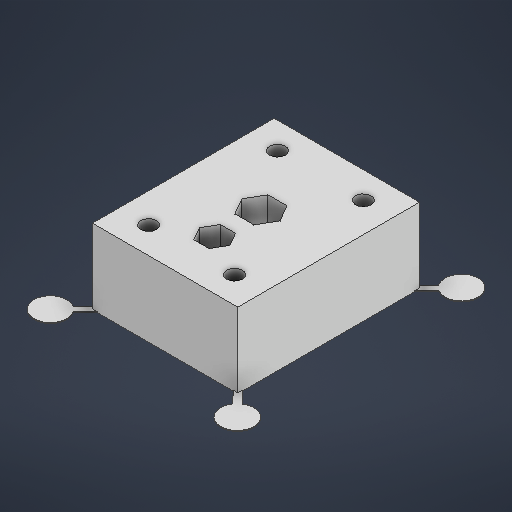
# Autodesk Inventor part: adapter-optical
Saved by Autodesk Inventor 2026.2 (Build 302298000, 298)
## iProperties
Created: 2026-05-22
Part Number: adapter-optical
Material: Generic
Document SubType Name: Modeling
Designer: mayhe
Density: 1 g/cm^3
Appearance: Default
Mass: 51.2124 g
Surface Area: 118.535 cm^2
Volume: 51.2124 cm^3
Author: mayhe
Autodesk Inventor part; units mm, degrees
ref_plane "YZ Plane" through (0, 0, 0) normal (1, 0, 0) x (0, 1, 0)
ref_plane "XZ Plane" through (0, 0, 0) normal (0, 1, 0) x (-1, 0, 0)
ref_plane "XY Plane" through (0, 0, 0) normal (0, 0, 1) x (1, 0, 0)
sketch "Sketch1" plane through (0, 0, 0) normal (1, 0, 0) x (0, 1, 0)
  line L0 (11.35, 27.5) -> (-11.35, 27.5)
  line L1 (-11.35, 27.5) -> (-11.35, -27.5)
  line L2 (-11.35, -27.5) -> (11.35, -27.5)
  line L3 (11.35, -27.5) -> (11.35, 27.5)
  line L4 (11.35, 27.5) -> (-11.35, -27.5) construction
  line L5 (-11.35, 27.5) -> (11.35, -27.5) construction
  point P0 (0, 0)
  dimension "d0" = 22.7
  dimension "d1" = 55
  constraints: 12 end point, 2 midpoint, 2 parallel, 1 horizontal, 1 perpendicular
  measures "d0" distance of L2.end L1.end
  measures "d1" distance of L1.end L0.end
extrude "Extrusion1" add sketch "Sketch1" along normal mid plane 44
sketch "Sketch4" plane through (-22, -11.35, 19.5) normal (0, 1, 0) x (1, 0, 0)
  circle A0 centre (9, 39) radius 2.375
  line L0 (0, 47) -> (44, 47) projected
  line L1 (0, -8) -> (0, 47) projected
  circle A1 centre (35, 39) radius 2.375
  circle A2 centre (9, 0) radius 2.375
  circle A3 centre (35, 0) radius 2.375
  line L2 (44, -8) -> (0, -8) projected
  point P0 (22, 19.5)
  dimension "d23" = 4.75
  dimension "d24" = 8
  dimension "d25" = 9
  dimension "d28" = 26
  dimension "d31" = 39
  dimension "d69" = 8
  constraints: 4 centre point, 1 horizontal, 1 vertical, 6 other
  measures "d23" diameter of A0
  measures "d24" distance from line of L0 A0.centre
  measures "d25" distance from line of L1 A0.centre
  measures "d28" distance of A0.centre A1.centre
  measures "d31" distance of A0.centre A2.centre
  measures "d69" distance from line of L2 A2.centre
hole "Event Camera mounting bolts" at (13, -11.35, -19.5) at (-13, -11.35, -19.5) at (-13, -11.35, 19.5) at (13, -11.35, 19.5) direction (0, 1, 0) diameter 4.75 depth 22.7 tip angle 118 counterbore diameter 7.7 counterbore depth 3
sketch "Sketch5" plane through (-22, -11.35, -27.5) normal (0, -1, 0) x (1, 0, 0)
  circle A0 centre (22, 40) radius 2
  circle A1 centre (22, 26) radius 2.5
  line L0 (44, 55) -> (0, 55) projected
  point P0 (22, 27.5)
  dimension "d41" = 4
  dimension "d42" = 5
  dimension "d43" = 14
  dimension "d44" = 15
  constraints: 2 centre point
  measures "d41" diameter of A0
  measures "d42" diameter of A1
  measures "d43" distance of A0.centre A1.centre
  measures "d44" distance from line of L0 A0.centre
hole "Small Hole" at (0, -11.35, 12.5) direction (0, 1, 0) diameter 5.75 depth 22.7 tip angle 118
hole "Big Hole" at (0, -11.35, -1.5) direction (0, 1, 0) diameter 6.75 depth 22.7 tip angle 118
sketch "Sketch6" plane through (-22, 11.35, 27.5) normal (0, 1, 0) x (1, 0, 0)
  circle A0 centre (22, 29) radius 3.375 projected
  circle A1 centre (22, 29) radius 5
  circle A2 centre (22, 15) radius 2.875 projected
  circle A3 centre (22, 15) radius 4
  line L0 (19.1132, 24) -> (16.2265, 29)
  line L1 (16.2265, 29) -> (19.1132, 34)
  line L2 (19.1132, 34) -> (24.8868, 34)
  line L3 (24.8868, 34) -> (27.7735, 29)
  line L4 (27.7735, 29) -> (24.8868, 24)
  line L5 (24.8868, 24) -> (19.1132, 24)
  line L6 (19.689, 11.0009) -> (17.3812, 15.0019)
  line L7 (17.3812, 15.0019) -> (19.6922, 19.0009)
  line L8 (19.6922, 19.0009) -> (24.311, 18.9991)
  line L9 (24.311, 18.9991) -> (26.6188, 14.9981)
  line L10 (26.6188, 14.9981) -> (24.3078, 10.9991)
  line L11 (24.3078, 10.9991) -> (19.689, 11.0009)
  point P0 (22, 27.5)
  point P1 (22, 24)
  point P2 (21.9984, 11)
  dimension "d59" = 10
  dimension "d60" = 8
  constraints: 24 end point, 4 coincident, 2 midpoint, 1 vertical alignment, 31 other
extrude "Big Hole Nut" cut sketch "Sketch6" against normal blind 8.5668 contours A0 | A1 | A1 L3 L4 | A1 L2 L3 | L4 L5 A1 | A1 L1 L2 | L5 L0 A1 | A1 L0 L1
extrude "Small Hole Nut" cut sketch "Sketch6" against normal blind 6.9668 contours A2 | A3 | A3 L9 L10 | A3 L8 L9 | L10 L11 A3 | A3 L7 L8 | L11 L6 A3 | A3 L6 L7
sketch "Sketch8" plane through (22, 11.35, -27.5) normal (0, 0, -1) x (-1, 0, 0)
  line L0 (-7.9257, -5.0636) -> (51.9257, -5.0636) construction
  line L1 (51.9257, -5.0636) -> (51.9257, -17.6364) construction
  line L2 (51.9257, -17.6364) -> (-7.9257, -17.6364) construction
  line L3 (-7.9257, -17.6364) -> (-7.9257, -5.0636) construction
  line L4 (24.8868, 0) -> (19.1132, 0) projected
  line L5 (22, 0) -> (22, -22.7)
  line L6 (44, -22.7) -> (0, -22.7) projected
  line L7 (44, 0) -> (0, 0) projected
  line L8 (7.086, -7.396) -> (7.086, -4.221)
  line L9 (7.086, -4.221) -> (9.2318, -4.221)
  line L10 (9.2318, -4.221) -> (9.2318, -4.8257)
  line L11 (9.2318, -4.8257) -> (7.8785, -4.8257)
  line L12 (7.8785, -4.8257) -> (7.8785, -5.384)
  line L13 (7.8785, -5.384) -> (9.1263, -5.384)
  line L14 (9.1263, -5.384) -> (9.1263, -5.9887)
  line L15 (9.1263, -5.9887) -> (7.8785, -5.9887)
  line L16 (7.8785, -5.9887) -> (7.8785, -6.7914)
  line L17 (7.8785, -6.7914) -> (9.2318, -6.7914)
  line L18 (9.2318, -6.7914) -> (9.2318, -7.396)
  line L19 (9.2318, -7.396) -> (7.086, -7.396)
  line L20 (11.9694, -5.0006) -> (11.1101, -7.396)
  line L21 (11.1101, -7.396) -> (10.2944, -7.396)
  line L22 (10.2944, -7.396) -> (9.4428, -5.0006)
  line L23 (9.4428, -5.0006) -> (10.2275, -5.0006)
  line L24 (10.2275, -5.0006) -> (10.719, -6.583)
  line L25 (10.719, -6.583) -> (11.2001, -5.0006)
  line L26 (11.2001, -5.0006) -> (11.9694, -5.0006)
  spline S0 degree 2 poles (13.4823, -7.4604) (12.803, -7.4604) (12.0801, -6.812) (12.0801, -6.2125) knots 0 0 0 1 2 2 2
  spline S1 degree 2 poles (12.0801, -6.2125) (12.0801, -5.6259) (12.7542, -4.926) (13.3614, -4.926) knots 0 0 0 1 2 2 2
  spline S2 degree 2 poles (13.3614, -4.926) (13.9094, -4.926) (14.4652, -5.5204) (14.4652, -6.071) knots 0 0 0 1 2 2 2
  line L27 (14.4652, -6.071) -> (14.4652, -6.3411)
  line L28 (14.4652, -6.3411) -> (12.8262, -6.3411)
  spline S3 degree 2 poles (12.8262, -6.3411) (12.8365, -6.5084) (12.9574, -6.7297) (13.0552, -6.7966) knots 0 0 0 1 2 2 2
  spline S4 degree 2 poles (13.0552, -6.7966) (13.1504, -6.8635) (13.4077, -6.9201) (13.5595, -6.9201) knots 0 0 0 1 2 2 2
  spline S5 degree 2 poles (13.5595, -6.9201) (13.6881, -6.9201) (13.9403, -6.8635) (14.0458, -6.8146) knots 0 0 0 1 2 2 2
  spline S6 degree 2 poles (14.0458, -6.8146) (14.1384, -6.776) (14.2928, -6.6808) (14.3417, -6.6448) knots 0 0 0 1 2 2 2
  line L29 (14.3417, -6.6448) -> (14.4214, -6.6448)
  line L30 (14.4214, -6.6448) -> (14.4214, -7.2623)
  spline S7 degree 2 poles (14.4214, -7.2623) (14.3288, -7.2983) (14.1796, -7.36) (14.0458, -7.3909) knots 0 0 0 1 2 2 2
  spline S8 degree 2 poles (14.0458, -7.3909) (13.9248, -7.4244) (13.6676, -7.4604) (13.4823, -7.4604) knots 0 0 0 1 2 2 2
  spline S9 degree 2 poles (13.7293, -5.8909) (13.7242, -5.6542) (13.5158, -5.4046) (13.3022, -5.4046) knots 0 0 0 1 2 2 2
  spline S10 degree 2 poles (13.3022, -5.4046) (13.0835, -5.4046) (12.8365, -5.667) (12.8236, -5.8909) knots 0 0 0 1 2 2 2
  line L31 (12.8236, -5.8909) -> (13.7293, -5.8909)
  line L32 (17.0896, -7.396) -> (16.3383, -7.396)
  line L33 (16.3383, -7.396) -> (16.3383, -6.2099)
  spline S11 degree 2 poles (16.3383, -6.2099) (16.3383, -6.0633) (16.3151, -5.7751) (16.2842, -5.7082) knots 0 0 0 1 2 2 2
  spline S12 degree 2 poles (16.2842, -5.7082) (16.2456, -5.6259) (16.1016, -5.5564) (15.978, -5.5564) knots 0 0 0 1 2 2 2
  spline S13 degree 2 poles (15.978, -5.5564) (15.888, -5.5564) (15.7002, -5.6259) (15.5947, -5.7005) knots 0 0 0 1 2 2 2
  line L34 (15.5947, -5.7005) -> (15.5947, -7.396)
  line L35 (15.5947, -7.396) -> (14.8485, -7.396)
  line L36 (14.8485, -7.396) -> (14.8485, -5.0006)
  line L37 (14.8485, -5.0006) -> (15.5947, -5.0006)
  line L38 (15.5947, -5.0006) -> (15.5947, -5.2657)
  spline S14 degree 2 poles (15.5947, -5.2657) (15.7774, -5.1113) (16.1247, -4.9363) (16.3357, -4.9363) knots 0 0 0 1 2 2 2
  spline S15 degree 2 poles (16.3357, -4.9363) (16.701, -4.9363) (17.0896, -5.3995) (17.0896, -5.8369) knots 0 0 0 1 2 2 2
  line L39 (17.0896, -5.8369) -> (17.0896, -7.396)
  spline S16 degree 2 poles (18.5587, -7.4424) (18.1033, -7.4424) (17.6865, -7.0667) (17.6865, -6.6396) knots 0 0 0 1 2 2 2
  line L40 (17.6865, -6.6396) -> (17.6865, -5.5204)
  line L41 (17.6865, -5.5204) -> (17.4009, -5.5204)
  line L42 (17.4009, -5.5204) -> (17.4009, -5.0006)
  line L43 (17.4009, -5.0006) -> (17.6865, -5.0006)
  line L44 (17.6865, -5.0006) -> (17.6865, -4.3162)
  line L45 (17.6865, -4.3162) -> (18.4326, -4.3162)
  line L46 (18.4326, -4.3162) -> (18.4326, -5.0006)
  line L47 (18.4326, -5.0006) -> (19.153, -5.0006)
  line L48 (19.153, -5.0006) -> (19.153, -5.5204)
  line L49 (19.153, -5.5204) -> (18.4326, -5.5204)
  line L50 (18.4326, -5.5204) -> (18.4326, -6.372)
  spline S17 degree 2 poles (18.4326, -6.372) (18.4326, -6.4981) (18.4378, -6.6859) (18.4686, -6.7605) knots 0 0 0 1 2 2 2
  spline S18 degree 2 poles (18.4686, -6.7605) (18.4995, -6.8351) (18.6513, -6.9226) (18.7954, -6.9226) knots 0 0 0 1 2 2 2
  spline S19 degree 2 poles (18.7954, -6.9226) (18.8572, -6.9226) (19.0501, -6.8712) (19.0887, -6.8506) knots 0 0 0 1 2 2 2
  line L51 (19.0887, -6.8506) -> (19.153, -6.8506)
  line L52 (19.153, -6.8506) -> (19.153, -7.3755)
  spline S20 degree 2 poles (19.153, -7.3755) (19.0321, -7.4063) (18.7594, -7.4424) (18.5587, -7.4424) knots 0 0 0 1 2 2 2
  spline S21 degree 2 poles (22.1479, -7.4578) (21.4327, -7.4578) (20.5939, -6.5933) (20.5939, -5.8111) knots 0 0 0 1 2 2 2
  spline S22 degree 2 poles (20.5939, -5.8111) (20.5939, -5.0573) (21.4352, -4.1593) (22.1505, -4.1593) knots 0 0 0 1 2 2 2
  spline S23 degree 2 poles (22.1505, -4.1593) (22.3383, -4.1593) (22.6419, -4.203) (22.7809, -4.2391) knots 0 0 0 1 2 2 2
  spline S24 degree 2 poles (22.7809, -4.2391) (22.8889, -4.2725) (23.1437, -4.3831) (23.2234, -4.4243) knots 0 0 0 1 2 2 2
  line L53 (23.2234, -4.4243) -> (23.2234, -5.1808)
  line L54 (23.2234, -5.1808) -> (23.1437, -5.1808)
  spline S25 degree 2 poles (23.1437, -5.1808) (23.0845, -5.1293) (22.9095, -4.9852) (22.7989, -4.9183) knots 0 0 0 1 2 2 2
  spline S26 degree 2 poles (22.7989, -4.9183) (22.6883, -4.8488) (22.4232, -4.7536) (22.2766, -4.7536) knots 0 0 0 1 2 2 2
  spline S27 degree 2 poles (22.2766, -4.7536) (22.1042, -4.7536) (21.8186, -4.8617) (21.6874, -4.9981) knots 0 0 0 1 2 2 2
  spline S28 degree 2 poles (21.6874, -4.9981) (21.569, -5.119) (21.4172, -5.5332) (21.4172, -5.8137) knots 0 0 0 1 2 2 2
  spline S29 degree 2 poles (21.4172, -5.8137) (21.4172, -6.1096) (21.5742, -6.5135) (21.7028, -6.637) knots 0 0 0 1 2 2 2
  spline S30 degree 2 poles (21.7028, -6.637) (21.8263, -6.758) (22.1299, -6.8635) (22.2817, -6.8635) knots 0 0 0 1 2 2 2
  spline S31 degree 2 poles (22.2817, -6.8635) (22.4387, -6.8635) (22.7243, -6.758) (22.8221, -6.6936) knots 0 0 0 1 2 2 2
  spline S32 degree 2 poles (22.8221, -6.6936) (22.9301, -6.6293) (23.0922, -6.4929) (23.1514, -6.4389) knots 0 0 0 1 2 2 2
  line L55 (23.1514, -6.4389) -> (23.2234, -6.4389)
  line L56 (23.2234, -6.4389) -> (23.2234, -7.1851)
  spline S33 degree 2 poles (23.2234, -7.1851) (23.136, -7.2262) (22.907, -7.3292) (22.7835, -7.3652) knots 0 0 0 1 2 2 2
  spline S34 degree 2 poles (22.7835, -7.3652) (22.6342, -7.4115) (22.3744, -7.4578) (22.1479, -7.4578) knots 0 0 0 1 2 2 2
  spline S35 degree 2 poles (24.9705, -7.1413) (24.8933, -7.2057) (24.7723, -7.3086) (24.6694, -7.36) knots 0 0 0 1 2 2 2
  spline S36 degree 2 poles (24.6694, -7.36) (24.5691, -7.4089) (24.3787, -7.4604) (24.2089, -7.4604) knots 0 0 0 1 2 2 2
  spline S37 degree 2 poles (24.2089, -7.4604) (23.8898, -7.4604) (23.4704, -7.0333) (23.4704, -6.7091) knots 0 0 0 1 2 2 2
  spline S38 degree 2 poles (23.4704, -6.7091) (23.4704, -6.4441) (23.684, -6.1147) (23.8847, -6.0195) knots 0 0 0 1 2 2 2
  spline S39 degree 2 poles (23.8847, -6.0195) (24.0879, -5.9218) (24.6514, -5.8446) (24.9756, -5.824) knots 0 0 0 1 2 2 2
  line L57 (24.9756, -5.824) -> (24.9756, -5.8111)
  spline S40 degree 2 poles (24.9756, -5.8111) (24.9756, -5.613) (24.6823, -5.4612) (24.389, -5.4612) knots 0 0 0 1 2 2 2
  spline S41 degree 2 poles (24.389, -5.4612) (24.2577, -5.4612) (23.9027, -5.5564) (23.7354, -5.631) knots 0 0 0 1 2 2 2
  line L58 (23.7354, -5.631) -> (23.6711, -5.631)
  line L59 (23.6711, -5.631) -> (23.6711, -5.0521)
  spline S42 degree 2 poles (23.6711, -5.0521) (23.7818, -5.0212) (24.2758, -4.9338) (24.5279, -4.9338) knots 0 0 0 1 2 2 2
  spline S43 degree 2 poles (24.5279, -4.9338) (25.1454, -4.9338) (25.7115, -5.3454) (25.7115, -5.7674) knots 0 0 0 1 2 2 2
  line L60 (25.7115, -5.7674) -> (25.7115, -7.396)
  line L61 (25.7115, -7.396) -> (24.9705, -7.396)
  line L62 (24.9705, -7.396) -> (24.9705, -7.1413)
  line L63 (24.9705, -6.7708) -> (24.9705, -6.2742)
  spline S44 degree 2 poles (24.9705, -6.2742) (24.7801, -6.2923) (24.5459, -6.3206) (24.4327, -6.3617) knots 0 0 0 1 2 2 2
  spline S45 degree 2 poles (24.4327, -6.3617) (24.3324, -6.3952) (24.2243, -6.5341) (24.2243, -6.6473) knots 0 0 0 1 2 2 2
  spline S46 degree 2 poles (24.2243, -6.6473) (24.2243, -6.8146) (24.407, -6.9406) (24.5845, -6.9406) knots 0 0 0 1 2 2 2
  spline S47 degree 2 poles (24.5845, -6.9406) (24.6823, -6.9406) (24.8881, -6.8506) (24.9705, -6.7708) knots 0 0 0 1 2 2 2
  line L64 (29.1232, -7.396) -> (29.1232, -6.1996)
  spline S48 degree 2 poles (29.1232, -6.1996) (29.1232, -6.0221) (29.1103, -5.7802) (29.0794, -5.7031) knots 0 0 0 1 2 2 2
  spline S49 degree 2 poles (29.0794, -5.7031) (29.046, -5.6259) (28.9122, -5.5564) (28.7913, -5.5564) knots 0 0 0 1 2 2 2
  spline S50 degree 2 poles (28.7913, -5.5564) (28.7064, -5.5564) (28.5417, -5.631) (28.4439, -5.7005) knots 0 0 0 1 2 2 2
  line L65 (28.4439, -5.7005) -> (28.4439, -7.396)
  line L66 (28.4439, -7.396) -> (27.6926, -7.396)
  line L67 (27.6926, -7.396) -> (27.6926, -6.1996)
  spline S51 degree 2 poles (27.6926, -6.1996) (27.6926, -6.0247) (27.6772, -5.7802) (27.6463, -5.7031) knots 0 0 0 1 2 2 2
  spline S52 degree 2 poles (27.6463, -5.7031) (27.6129, -5.6259) (27.4791, -5.5564) (27.3581, -5.5564) knots 0 0 0 1 2 2 2
  spline S53 degree 2 poles (27.3581, -5.5564) (27.2681, -5.5564) (27.0905, -5.6413) (27.0082, -5.7005) knots 0 0 0 1 2 2 2
  line L68 (27.0082, -5.7005) -> (27.0082, -7.396)
  line L69 (27.0082, -7.396) -> (26.2621, -7.396)
  line L70 (26.2621, -7.396) -> (26.2621, -5.0006)
  line L71 (26.2621, -5.0006) -> (27.0082, -5.0006)
  line L72 (27.0082, -5.0006) -> (27.0082, -5.2657)
  spline S54 degree 2 poles (27.0082, -5.2657) (27.1909, -5.1113) (27.5177, -4.9363) (27.7209, -4.9363) knots 0 0 0 1 2 2 2
  spline S55 degree 2 poles (27.7209, -4.9363) (27.9396, -4.9363) (28.2741, -5.1447) (28.3616, -5.3531) knots 0 0 0 1 2 2 2
  spline S56 degree 2 poles (28.3616, -5.3531) (28.5751, -5.1525) (28.9559, -4.9363) (29.1515, -4.9363) knots 0 0 0 1 2 2 2
  spline S57 degree 2 poles (29.1515, -4.9363) (29.3187, -4.9363) (29.5837, -5.0418) (29.6738, -5.1499) knots 0 0 0 1 2 2 2
  spline S58 degree 2 poles (29.6738, -5.1499) (29.7741, -5.2657) (29.8745, -5.5821) (29.8745, -5.8369) knots 0 0 0 1 2 2 2
  line L73 (29.8745, -5.8369) -> (29.8745, -7.396)
  line L74 (29.8745, -7.396) -> (29.1232, -7.396)
  spline S59 degree 2 poles (31.6549, -7.4604) (30.9757, -7.4604) (30.2527, -6.812) (30.2527, -6.2125) knots 0 0 0 1 2 2 2
  spline S60 degree 2 poles (30.2527, -6.2125) (30.2527, -5.6259) (30.9268, -4.926) (31.534, -4.926) knots 0 0 0 1 2 2 2
  spline S61 degree 2 poles (31.534, -4.926) (32.082, -4.926) (32.6378, -5.5204) (32.6378, -6.071) knots 0 0 0 1 2 2 2
  line L75 (32.6378, -6.071) -> (32.6378, -6.3411)
  line L76 (32.6378, -6.3411) -> (30.9988, -6.3411)
  spline S62 degree 2 poles (30.9988, -6.3411) (31.0091, -6.5084) (31.1301, -6.7297) (31.2278, -6.7966) knots 0 0 0 1 2 2 2
  spline S63 degree 2 poles (31.2278, -6.7966) (31.323, -6.8635) (31.5803, -6.9201) (31.7321, -6.9201) knots 0 0 0 1 2 2 2
  spline S64 degree 2 poles (31.7321, -6.9201) (31.8608, -6.9201) (32.1129, -6.8635) (32.2184, -6.8146) knots 0 0 0 1 2 2 2
  spline S65 degree 2 poles (32.2184, -6.8146) (32.311, -6.776) (32.4654, -6.6808) (32.5143, -6.6448) knots 0 0 0 1 2 2 2
  line L77 (32.5143, -6.6448) -> (32.5941, -6.6448)
  line L78 (32.5941, -6.6448) -> (32.5941, -7.2623)
  spline S66 degree 2 poles (32.5941, -7.2623) (32.5014, -7.2983) (32.3522, -7.36) (32.2184, -7.3909) knots 0 0 0 1 2 2 2
  spline S67 degree 2 poles (32.2184, -7.3909) (32.0975, -7.4244) (31.8402, -7.4604) (31.6549, -7.4604) knots 0 0 0 1 2 2 2
  spline S68 degree 2 poles (31.9019, -5.8909) (31.8968, -5.6542) (31.6884, -5.4046) (31.4748, -5.4046) knots 0 0 0 1 2 2 2
  spline S69 degree 2 poles (31.4748, -5.4046) (31.2561, -5.4046) (31.0091, -5.667) (30.9963, -5.8909) knots 0 0 0 1 2 2 2
  line L79 (30.9963, -5.8909) -> (31.9019, -5.8909)
  line L80 (34.6292, -5.7082) -> (34.5675, -5.7082)
  spline S70 degree 2 poles (34.5675, -5.7082) (34.5238, -5.6928) (34.3617, -5.6773) (34.2639, -5.6773) knots 0 0 0 1 2 2 2
  spline S71 degree 2 poles (34.2639, -5.6773) (34.1481, -5.6773) (33.8882, -5.7468) (33.7673, -5.7931) knots 0 0 0 1 2 2 2
  line L81 (33.7673, -5.7931) -> (33.7673, -7.396)
  line L82 (33.7673, -7.396) -> (33.0212, -7.396)
  line L83 (33.0212, -7.396) -> (33.0212, -5.0006)
  line L84 (33.0212, -5.0006) -> (33.7673, -5.0006)
  line L85 (33.7673, -5.0006) -> (33.7673, -5.3454)
  spline S72 degree 2 poles (33.7673, -5.3454) (33.8188, -5.2991) (33.9989, -5.155) (34.0735, -5.1113) knots 0 0 0 1 2 2 2
  spline S73 degree 2 poles (34.0735, -5.1113) (34.1558, -5.0624) (34.372, -4.9929) (34.4671, -4.9929) knots 0 0 0 1 2 2 2
  spline S74 degree 2 poles (34.4671, -4.9929) (34.5032, -4.9929) (34.5932, -4.9981) (34.6292, -5.0006) knots 0 0 0 1 2 2 2
  line L86 (34.6292, -5.0006) -> (34.6292, -5.7082)
  spline S75 degree 2 poles (36.2348, -7.1413) (36.1576, -7.2057) (36.0366, -7.3086) (35.9337, -7.36) knots 0 0 0 1 2 2 2
  spline S76 degree 2 poles (35.9337, -7.36) (35.8334, -7.4089) (35.643, -7.4604) (35.4732, -7.4604) knots 0 0 0 1 2 2 2
  spline S77 degree 2 poles (35.4732, -7.4604) (35.1541, -7.4604) (34.7347, -7.0333) (34.7347, -6.7091) knots 0 0 0 1 2 2 2
  spline S78 degree 2 poles (34.7347, -6.7091) (34.7347, -6.4441) (34.9483, -6.1147) (35.149, -6.0195) knots 0 0 0 1 2 2 2
  spline S79 degree 2 poles (35.149, -6.0195) (35.3522, -5.9218) (35.9157, -5.8446) (36.2399, -5.824) knots 0 0 0 1 2 2 2
  line L87 (36.2399, -5.824) -> (36.2399, -5.8111)
  spline S80 degree 2 poles (36.2399, -5.8111) (36.2399, -5.613) (35.9466, -5.4612) (35.6533, -5.4612) knots 0 0 0 1 2 2 2
  spline S81 degree 2 poles (35.6533, -5.4612) (35.5221, -5.4612) (35.167, -5.5564) (34.9997, -5.631) knots 0 0 0 1 2 2 2
  line L88 (34.9997, -5.631) -> (34.9354, -5.631)
  line L89 (34.9354, -5.631) -> (34.9354, -5.0521)
  spline S82 degree 2 poles (34.9354, -5.0521) (35.0461, -5.0212) (35.5401, -4.9338) (35.7922, -4.9338) knots 0 0 0 1 2 2 2
  spline S83 degree 2 poles (35.7922, -4.9338) (36.4097, -4.9338) (36.9758, -5.3454) (36.9758, -5.7674) knots 0 0 0 1 2 2 2
  line L90 (36.9758, -5.7674) -> (36.9758, -7.396)
  line L91 (36.9758, -7.396) -> (36.2348, -7.396)
  line L92 (36.2348, -7.396) -> (36.2348, -7.1413)
  line L93 (36.2348, -6.7708) -> (36.2348, -6.2742)
  spline S84 degree 2 poles (36.2348, -6.2742) (36.0444, -6.2923) (35.8102, -6.3206) (35.697, -6.3617) knots 0 0 0 1 2 2 2
  spline S85 degree 2 poles (35.697, -6.3617) (35.5967, -6.3952) (35.4886, -6.5341) (35.4886, -6.6473) knots 0 0 0 1 2 2 2
  spline S86 degree 2 poles (35.4886, -6.6473) (35.4886, -6.8146) (35.6713, -6.9406) (35.8488, -6.9406) knots 0 0 0 1 2 2 2
  spline S87 degree 2 poles (35.8488, -6.9406) (35.9466, -6.9406) (36.1524, -6.8506) (36.2348, -6.7708) knots 0 0 0 1 2 2 2
  line L94 (13.2868, -12.6236) -> (14.3597, -9.4486)
  line L95 (14.3597, -9.4486) -> (15.2293, -9.4486)
  line L96 (15.2293, -9.4486) -> (16.3022, -12.6236)
  line L97 (16.3022, -12.6236) -> (15.4815, -12.6236)
  line L98 (15.4815, -12.6236) -> (15.2834, -11.9752)
  line L99 (15.2834, -11.9752) -> (14.2851, -11.9752)
  line L100 (14.2851, -11.9752) -> (14.0844, -12.6236)
  line L101 (14.0844, -12.6236) -> (13.2868, -12.6236)
  line L102 (15.1084, -11.3989) -> (14.7842, -10.3491)
  line L103 (14.7842, -10.3491) -> (14.4574, -11.3989)
  line L104 (14.4574, -11.3989) -> (15.1084, -11.3989)
  line L105 (18.7517, -12.6236) -> (18.0055, -12.6236)
  line L106 (18.0055, -12.6236) -> (18.0055, -12.374)
  spline S88 degree 2 poles (18.0055, -12.374) (17.9335, -12.4332) (17.7482, -12.5696) (17.6762, -12.6056) knots 0 0 0 1 2 2 2
  spline S89 degree 2 poles (17.6762, -12.6056) (17.5887, -12.6468) (17.4137, -12.6905) (17.2928, -12.6905) knots 0 0 0 1 2 2 2
  spline S90 degree 2 poles (17.2928, -12.6905) (16.8837, -12.6905) (16.4052, -12.0112) (16.4052, -11.4452) knots 0 0 0 1 2 2 2
  spline S91 degree 2 poles (16.4052, -11.4452) (16.4052, -11.1313) (16.5673, -10.6707) (16.7088, -10.5009) knots 0 0 0 1 2 2 2
  spline S92 degree 2 poles (16.7088, -10.5009) (16.84, -10.344) (17.2105, -10.1639) (17.4163, -10.1639) knots 0 0 0 1 2 2 2
  spline S93 degree 2 poles (17.4163, -10.1639) (17.6041, -10.1639) (17.846, -10.2436) (18.0055, -10.326) knots 0 0 0 1 2 2 2
  line L107 (18.0055, -10.326) -> (18.0055, -9.3071)
  line L108 (18.0055, -9.3071) -> (18.7517, -9.3071)
  line L109 (18.7517, -9.3071) -> (18.7517, -12.6236)
  line L110 (18.0055, -11.9649) -> (18.0055, -10.7891)
  spline S94 degree 2 poles (18.0055, -10.7891) (17.9515, -10.7608) (17.7714, -10.7248) (17.7071, -10.7248) knots 0 0 0 1 2 2 2
  spline S95 degree 2 poles (17.7071, -10.7248) (17.4395, -10.7248) (17.1693, -11.1004) (17.1693, -11.4375) knots 0 0 0 1 2 2 2
  spline S96 degree 2 poles (17.1693, -11.4375) (17.1693, -11.7925) (17.3854, -12.109) (17.6247, -12.109) knots 0 0 0 1 2 2 2
  spline S97 degree 2 poles (17.6247, -12.109) (17.7225, -12.109) (17.9232, -12.0318) (18.0055, -11.9649) knots 0 0 0 1 2 2 2
  spline S98 degree 2 poles (20.6428, -12.3689) (20.5656, -12.4332) (20.4447, -12.5361) (20.3417, -12.5876) knots 0 0 0 1 2 2 2
  spline S99 degree 2 poles (20.3417, -12.5876) (20.2414, -12.6365) (20.051, -12.6879) (19.8812, -12.6879) knots 0 0 0 1 2 2 2
  spline S100 degree 2 poles (19.8812, -12.6879) (19.5621, -12.6879) (19.1428, -12.2608) (19.1428, -11.9366) knots 0 0 0 1 2 2 2
  spline S101 degree 2 poles (19.1428, -11.9366) (19.1428, -11.6716) (19.3563, -11.3423) (19.557, -11.2471) knots 0 0 0 1 2 2 2
  spline S102 degree 2 poles (19.557, -11.2471) (19.7603, -11.1493) (20.3237, -11.0721) (20.6479, -11.0515) knots 0 0 0 1 2 2 2
  line L111 (20.6479, -11.0515) -> (20.6479, -11.0387)
  spline S103 degree 2 poles (20.6479, -11.0387) (20.6479, -10.8406) (20.3546, -10.6888) (20.0613, -10.6888) knots 0 0 0 1 2 2 2
  spline S104 degree 2 poles (20.0613, -10.6888) (19.9301, -10.6888) (19.575, -10.784) (19.4078, -10.8586) knots 0 0 0 1 2 2 2
  line L112 (19.4078, -10.8586) -> (19.3434, -10.8586)
  line L113 (19.3434, -10.8586) -> (19.3434, -10.2797)
  spline S105 degree 2 poles (19.3434, -10.2797) (19.4541, -10.2488) (19.9481, -10.1613) (20.2002, -10.1613) knots 0 0 0 1 2 2 2
  spline S106 degree 2 poles (20.2002, -10.1613) (20.8177, -10.1613) (21.3838, -10.573) (21.3838, -10.9949) knots 0 0 0 1 2 2 2
  line L114 (21.3838, -10.9949) -> (21.3838, -12.6236)
  line L115 (21.3838, -12.6236) -> (20.6428, -12.6236)
  line L116 (20.6428, -12.6236) -> (20.6428, -12.3689)
  line L117 (20.6428, -11.9984) -> (20.6428, -11.5018)
  spline S107 degree 2 poles (20.6428, -11.5018) (20.4524, -11.5198) (20.2182, -11.5481) (20.105, -11.5893) knots 0 0 0 1 2 2 2
  spline S108 degree 2 poles (20.105, -11.5893) (20.0047, -11.6227) (19.8966, -11.7617) (19.8966, -11.8749) knots 0 0 0 1 2 2 2
  spline S109 degree 2 poles (19.8966, -11.8749) (19.8966, -12.0421) (20.0793, -12.1682) (20.2568, -12.1682) knots 0 0 0 1 2 2 2
  spline S110 degree 2 poles (20.2568, -12.1682) (20.3546, -12.1682) (20.5604, -12.0781) (20.6428, -11.9984) knots 0 0 0 1 2 2 2
  spline S111 degree 2 poles (24.2835, -11.3937) (24.2835, -11.9675) (23.702, -12.6699) (23.2749, -12.6699) knots 0 0 0 1 2 2 2
  spline S112 degree 2 poles (23.2749, -12.6699) (23.0974, -12.6699) (22.8323, -12.5902) (22.6831, -12.5027) knots 0 0 0 1 2 2 2
  line L118 (22.6831, -12.5027) -> (22.6831, -13.501)
  line L119 (22.6831, -13.501) -> (21.937, -13.501)
  line L120 (21.937, -13.501) -> (21.937, -10.2282)
  line L121 (21.937, -10.2282) -> (22.6831, -10.2282)
  line L122 (22.6831, -10.2282) -> (22.6831, -10.4803)
  spline S113 degree 2 poles (22.6831, -10.4803) (22.8478, -10.3388) (23.1874, -10.1639) (23.4113, -10.1639) knots 0 0 0 1 2 2 2
  spline S114 degree 2 poles (23.4113, -10.1639) (23.8281, -10.1639) (24.2835, -10.8251) (24.2835, -11.3937) knots 0 0 0 1 2 2 2
  spline S115 degree 2 poles (23.5193, -11.4092) (23.5193, -11.0593) (23.3032, -10.7454) (23.0768, -10.7454) knots 0 0 0 1 2 2 2
  spline S116 degree 2 poles (23.0768, -10.7454) (22.9764, -10.7454) (22.7783, -10.8097) (22.6831, -10.874) knots 0 0 0 1 2 2 2
  line L123 (22.6831, -10.874) -> (22.6831, -12.0756)
  spline S117 degree 2 poles (22.6831, -12.0756) (22.7423, -12.1013) (22.8864, -12.1219) (22.9841, -12.1219) knots 0 0 0 1 2 2 2
  spline S118 degree 2 poles (22.9841, -12.1219) (23.2543, -12.1219) (23.5193, -11.7668) (23.5193, -11.4092) knots 0 0 0 1 2 2 2
  spline S119 degree 2 poles (25.6008, -12.6699) (25.1454, -12.6699) (24.7286, -12.2943) (24.7286, -11.8672) knots 0 0 0 1 2 2 2
  line L124 (24.7286, -11.8672) -> (24.7286, -10.7479)
  line L125 (24.7286, -10.7479) -> (24.443, -10.7479)
  line L126 (24.443, -10.7479) -> (24.443, -10.2282)
  line L127 (24.443, -10.2282) -> (24.7286, -10.2282)
  line L128 (24.7286, -10.2282) -> (24.7286, -9.5438)
  line L129 (24.7286, -9.5438) -> (25.4747, -9.5438)
  line L130 (25.4747, -9.5438) -> (25.4747, -10.2282)
  line L131 (25.4747, -10.2282) -> (26.1952, -10.2282)
  line L132 (26.1952, -10.2282) -> (26.1952, -10.7479)
  line L133 (26.1952, -10.7479) -> (25.4747, -10.7479)
  line L134 (25.4747, -10.7479) -> (25.4747, -11.5996)
  spline S120 degree 2 poles (25.4747, -11.5996) (25.4747, -11.7256) (25.4799, -11.9135) (25.5108, -11.9881) knots 0 0 0 1 2 2 2
  spline S121 degree 2 poles (25.5108, -11.9881) (25.5416, -12.0627) (25.6934, -12.1502) (25.8375, -12.1502) knots 0 0 0 1 2 2 2
  spline S122 degree 2 poles (25.8375, -12.1502) (25.8993, -12.1502) (26.0923, -12.0987) (26.1308, -12.0781) knots 0 0 0 1 2 2 2
  line L135 (26.1308, -12.0781) -> (26.1952, -12.0781)
  line L136 (26.1952, -12.0781) -> (26.1952, -12.603)
  spline S123 degree 2 poles (26.1952, -12.603) (26.0742, -12.6339) (25.8015, -12.6699) (25.6008, -12.6699) knots 0 0 0 1 2 2 2
  spline S124 degree 2 poles (27.7261, -12.6879) (27.0468, -12.6879) (26.3238, -12.0395) (26.3238, -11.4401) knots 0 0 0 1 2 2 2
  spline S125 degree 2 poles (26.3238, -11.4401) (26.3238, -10.8534) (26.9979, -10.1536) (27.6051, -10.1536) knots 0 0 0 1 2 2 2
  spline S126 degree 2 poles (27.6051, -10.1536) (28.1532, -10.1536) (28.7089, -10.7479) (28.7089, -11.2985) knots 0 0 0 1 2 2 2
  line L137 (28.7089, -11.2985) -> (28.7089, -11.5687)
  line L138 (28.7089, -11.5687) -> (27.07, -11.5687)
  spline S127 degree 2 poles (27.07, -11.5687) (27.0803, -11.7359) (27.2012, -11.9572) (27.299, -12.0241) knots 0 0 0 1 2 2 2
  spline S128 degree 2 poles (27.299, -12.0241) (27.3942, -12.091) (27.6514, -12.1476) (27.8033, -12.1476) knots 0 0 0 1 2 2 2
  spline S129 degree 2 poles (27.8033, -12.1476) (27.9319, -12.1476) (28.184, -12.091) (28.2895, -12.0421) knots 0 0 0 1 2 2 2
  spline S130 degree 2 poles (28.2895, -12.0421) (28.3822, -12.0035) (28.5365, -11.9083) (28.5854, -11.8723) knots 0 0 0 1 2 2 2
  line L139 (28.5854, -11.8723) -> (28.6652, -11.8723)
  line L140 (28.6652, -11.8723) -> (28.6652, -12.4898)
  spline S131 degree 2 poles (28.6652, -12.4898) (28.5726, -12.5258) (28.4233, -12.5876) (28.2895, -12.6185) knots 0 0 0 1 2 2 2
  spline S132 degree 2 poles (28.2895, -12.6185) (28.1686, -12.6519) (27.9113, -12.6879) (27.7261, -12.6879) knots 0 0 0 1 2 2 2
  spline S133 degree 2 poles (27.9731, -11.1184) (27.9679, -10.8817) (27.7595, -10.6322) (27.546, -10.6322) knots 0 0 0 1 2 2 2
  spline S134 degree 2 poles (27.546, -10.6322) (27.3273, -10.6322) (27.0803, -10.8946) (27.0674, -11.1184) knots 0 0 0 1 2 2 2
  line L141 (27.0674, -11.1184) -> (27.9731, -11.1184)
  line L142 (30.7004, -10.9358) -> (30.6386, -10.9358)
  spline S135 degree 2 poles (30.6386, -10.9358) (30.5949, -10.9203) (30.4328, -10.9049) (30.335, -10.9049) knots 0 0 0 1 2 2 2
  spline S136 degree 2 poles (30.335, -10.9049) (30.2192, -10.9049) (29.9594, -10.9744) (29.8384, -11.0207) knots 0 0 0 1 2 2 2
  line L143 (29.8384, -11.0207) -> (29.8384, -12.6236)
  line L144 (29.8384, -12.6236) -> (29.0923, -12.6236)
  line L145 (29.0923, -12.6236) -> (29.0923, -10.2282)
  line L146 (29.0923, -10.2282) -> (29.8384, -10.2282)
  line L147 (29.8384, -10.2282) -> (29.8384, -10.573)
  spline S137 degree 2 poles (29.8384, -10.573) (29.8899, -10.5267) (30.07, -10.3826) (30.1446, -10.3388) knots 0 0 0 1 2 2 2
  spline S138 degree 2 poles (30.1446, -10.3388) (30.227, -10.29) (30.4431, -10.2205) (30.5383, -10.2205) knots 0 0 0 1 2 2 2
  spline S139 degree 2 poles (30.5383, -10.2205) (30.5743, -10.2205) (30.6644, -10.2256) (30.7004, -10.2282) knots 0 0 0 1 2 2 2
  line L148 (30.7004, -10.2282) -> (30.7004, -10.9358)
  spline S140 degree 2 poles (13.7743, -16.7705) (13.7743, -17.2722) (13.1388, -17.9181) (12.5831, -17.9181) knots 0 0 0 1 2 2 2
  spline S141 degree 2 poles (12.5831, -17.9181) (12.3052, -17.9181) (11.8704, -17.7585) (11.7186, -17.6016) knots 0 0 0 1 2 2 2
  spline S142 degree 2 poles (11.7186, -17.6016) (11.5385, -17.4189) (11.3455, -16.84) (11.3455, -16.436) knots 0 0 0 1 2 2 2
  spline S143 degree 2 poles (11.3455, -16.436) (11.3455, -16.0192) (11.5256, -15.3708) (11.7288, -15.1213) knots 0 0 0 1 2 2 2
  spline S144 degree 2 poles (11.7288, -15.1213) (11.9218, -14.8846) (12.5496, -14.617) (12.9793, -14.617) knots 0 0 0 1 2 2 2
  spline S145 degree 2 poles (12.9793, -14.617) (13.1362, -14.617) (13.4501, -14.6581) (13.5067, -14.671) knots 0 0 0 1 2 2 2
  line L149 (13.5067, -14.671) -> (13.5067, -15.2937)
  line L150 (13.5067, -15.2937) -> (13.4501, -15.2937)
  spline S146 degree 2 poles (13.4501, -15.2937) (13.3935, -15.2654) (13.1362, -15.1959) (12.9716, -15.1959) knots 0 0 0 1 2 2 2
  spline S147 degree 2 poles (12.9716, -15.1959) (12.5985, -15.1959) (12.192, -15.5895) (12.1431, -15.9549) knots 0 0 0 1 2 2 2
  spline S148 degree 2 poles (12.1431, -15.9549) (12.3, -15.8546) (12.6217, -15.7362) (12.8249, -15.7362) knots 0 0 0 1 2 2 2
  spline S149 degree 2 poles (12.8249, -15.7362) (12.9973, -15.7362) (13.2983, -15.8288) (13.4141, -15.9163) knots 0 0 0 1 2 2 2
  spline S150 degree 2 poles (13.4141, -15.9163) (13.5788, -16.0424) (13.7743, -16.4515) (13.7743, -16.7705) knots 0 0 0 1 2 2 2
  spline S151 degree 2 poles (12.8455, -17.2491) (12.9073, -17.1719) (12.9741, -16.9918) (12.9741, -16.8091) knots 0 0 0 1 2 2 2
  spline S152 degree 2 poles (12.9741, -16.8091) (12.9741, -16.6547) (12.897, -16.4541) (12.8275, -16.3949) knots 0 0 0 1 2 2 2
  spline S153 degree 2 poles (12.8275, -16.3949) (12.7555, -16.3331) (12.5779, -16.2894) (12.4776, -16.2894) knots 0 0 0 1 2 2 2
  spline S154 degree 2 poles (12.4776, -16.2894) (12.3927, -16.2894) (12.2177, -16.3331) (12.1405, -16.364) knots 0 0 0 1 2 2 2
  spline S155 degree 2 poles (12.1405, -16.364) (12.1405, -16.3846) (12.1354, -16.4824) (12.1354, -16.557) knots 0 0 0 1 2 2 2
  spline S156 degree 2 poles (12.1354, -16.557) (12.1354, -16.8323) (12.2306, -17.1642) (12.3052, -17.2491) knots 0 0 0 1 2 2 2
  spline S157 degree 2 poles (12.3052, -17.2491) (12.3592, -17.3186) (12.5033, -17.3777) (12.5805, -17.3777) knots 0 0 0 1 2 2 2
  spline S158 degree 2 poles (12.5805, -17.3777) (12.6448, -17.3777) (12.794, -17.3134) (12.8455, -17.2491) knots 0 0 0 1 2 2 2
  line L151 (16.0462, -14.5346) -> (14.7829, -18.5407)
  line L152 (14.7829, -18.5407) -> (14.1706, -18.5407)
  line L153 (14.1706, -18.5407) -> (15.4313, -14.5346)
  line L154 (15.4313, -14.5346) -> (16.0462, -14.5346)
  spline S159 degree 2 poles (19.0849, -16.9686) (19.0849, -17.1719) (18.9151, -17.5244) (18.753, -17.653) knots 0 0 0 1 2 2 2
  spline S160 degree 2 poles (18.753, -17.653) (18.5909, -17.7817) (18.1252, -17.9258) (17.8241, -17.9258) knots 0 0 0 1 2 2 2
  spline S161 degree 2 poles (17.8241, -17.9258) (17.5025, -17.9258) (17.0214, -17.7791) (16.867, -17.653) knots 0 0 0 1 2 2 2
  spline S162 degree 2 poles (16.867, -17.653) (16.7152, -17.527) (16.5711, -17.1848) (16.5711, -16.9944) knots 0 0 0 1 2 2 2
  spline S163 degree 2 poles (16.5711, -16.9944) (16.5711, -16.7216) (16.8721, -16.3589) (17.1577, -16.2379) knots 0 0 0 1 2 2 2
  line L155 (17.1577, -16.2379) -> (17.1577, -16.2251)
  spline S164 degree 2 poles (17.1577, -16.2251) (16.8773, -16.0887) (16.656, -15.7002) (16.656, -15.4609) knots 0 0 0 1 2 2 2
  spline S165 degree 2 poles (16.656, -15.4609) (16.656, -15.2859) (16.8104, -14.9798) (16.9622, -14.8588) knots 0 0 0 1 2 2 2
  spline S166 degree 2 poles (16.9622, -14.8588) (17.1089, -14.7431) (17.554, -14.6041) (17.8318, -14.6041) knots 0 0 0 1 2 2 2
  spline S167 degree 2 poles (17.8318, -14.6041) (18.1252, -14.6041) (18.5626, -14.7302) (18.7041, -14.8331) knots 0 0 0 1 2 2 2
  spline S168 degree 2 poles (18.7041, -14.8331) (18.8482, -14.936) (19.0025, -15.2345) (19.0025, -15.4069) knots 0 0 0 1 2 2 2
  spline S169 degree 2 poles (19.0025, -15.4069) (19.0025, -15.6333) (18.7401, -15.9961) (18.4699, -16.1221) knots 0 0 0 1 2 2 2
  line L156 (18.4699, -16.1221) -> (18.4699, -16.1324)
  spline S170 degree 2 poles (18.4699, -16.1324) (18.7864, -16.2611) (19.0849, -16.6779) (19.0849, -16.9686) knots 0 0 0 1 2 2 2
  spline S171 degree 2 poles (18.2975, -17.0021) (18.2975, -16.8451) (18.1638, -16.6805) (17.9476, -16.575) knots 0 0 0 1 2 2 2
  spline S172 degree 2 poles (17.9476, -16.575) (17.8859, -16.5467) (17.6517, -16.4566) (17.5617, -16.418) knots 0 0 0 1 2 2 2
  spline S173 degree 2 poles (17.5617, -16.418) (17.4794, -16.5004) (17.3481, -16.7474) (17.3481, -16.894) knots 0 0 0 1 2 2 2
  spline S174 degree 2 poles (17.3481, -16.894) (17.3481, -17.1153) (17.6312, -17.3803) (17.8602, -17.3803) knots 0 0 0 1 2 2 2
  spline S175 degree 2 poles (17.8602, -17.3803) (17.9245, -17.3803) (18.084, -17.3391) (18.1457, -17.298) knots 0 0 0 1 2 2 2
  spline S176 degree 2 poles (18.1457, -17.298) (18.2152, -17.2491) (18.2975, -17.1153) (18.2975, -17.0021) knots 0 0 0 1 2 2 2
  spline S177 degree 2 poles (18.2281, -15.4995) (18.2281, -15.3374) (18.0145, -15.1444) (17.8318, -15.1444) knots 0 0 0 1 2 2 2
  spline S178 degree 2 poles (17.8318, -15.1444) (17.6569, -15.1444) (17.4433, -15.3194) (17.4433, -15.448) knots 0 0 0 1 2 2 2
  spline S179 degree 2 poles (17.4433, -15.448) (17.4433, -15.5741) (17.572, -15.7311) (17.7083, -15.7954) knots 0 0 0 1 2 2 2
  spline S180 degree 2 poles (17.7083, -15.7954) (17.7675, -15.8263) (17.9322, -15.8906) (18.0686, -15.942) knots 0 0 0 1 2 2 2
  spline S181 degree 2 poles (18.0686, -15.942) (18.1509, -15.834) (18.2281, -15.6307) (18.2281, -15.4995) knots 0 0 0 1 2 2 2
  line L157 (21.3465, -14.5346) -> (20.0832, -18.5407)
  line L158 (20.0832, -18.5407) -> (19.4708, -18.5407)
  line L159 (19.4708, -18.5407) -> (20.7315, -14.5346)
  line L160 (20.7315, -14.5346) -> (21.3465, -14.5346)
  line L161 (24.3928, -17.8512) -> (22.0592, -17.8512)
  line L162 (22.0592, -17.8512) -> (22.0592, -17.334)
  spline S182 degree 2 poles (22.0592, -17.334) (22.3551, -17.0973) (22.8285, -16.6805) (23.006, -16.4926) knots 0 0 0 1 2 2 2
  spline S183 degree 2 poles (23.006, -16.4926) (23.2402, -16.2482) (23.4486, -15.8751) (23.4486, -15.6796) knots 0 0 0 1 2 2 2
  spline S184 degree 2 poles (23.4486, -15.6796) (23.4486, -15.4583) (23.1835, -15.2216) (22.9468, -15.2216) knots 0 0 0 1 2 2 2
  spline S185 degree 2 poles (22.9468, -15.2216) (22.8259, -15.2216) (22.6098, -15.2808) (22.4991, -15.3271) knots 0 0 0 1 2 2 2
  spline S186 degree 2 poles (22.4991, -15.3271) (22.3911, -15.376) (22.2367, -15.4789) (22.1981, -15.5046) knots 0 0 0 1 2 2 2
  line L163 (22.1981, -15.5046) -> (22.1364, -15.5046)
  line L164 (22.1364, -15.5046) -> (22.1364, -14.8125)
  spline S187 degree 2 poles (22.1364, -14.8125) (22.2702, -14.7482) (22.8413, -14.6144) (23.1064, -14.6144) knots 0 0 0 1 2 2 2
  spline S188 degree 2 poles (23.1064, -14.6144) (23.6724, -14.6144) (24.2539, -15.1187) (24.2539, -15.5741) knots 0 0 0 1 2 2 2
  spline S189 degree 2 poles (24.2539, -15.5741) (24.2539, -15.8546) (23.9889, -16.3949) (23.6827, -16.7036) knots 0 0 0 1 2 2 2
  spline S190 degree 2 poles (23.6827, -16.7036) (23.4897, -16.894) (23.1269, -17.1899) (23.0472, -17.2517) knots 0 0 0 1 2 2 2
  line L165 (23.0472, -17.2517) -> (24.3928, -17.2517)
  line L166 (24.3928, -17.2517) -> (24.3928, -17.8512)
  spline S191 degree 2 poles (27.133, -16.2637) (27.133, -16.6753) (27.0018, -17.2928) (26.8551, -17.5012) knots 0 0 0 1 2 2 2
  spline S192 degree 2 poles (26.8551, -17.5012) (26.711, -17.7071) (26.2453, -17.9181) (25.9109, -17.9181) knots 0 0 0 1 2 2 2
  spline S193 degree 2 poles (25.9109, -17.9181) (25.5738, -17.9181) (25.1107, -17.7071) (24.964, -17.4961) knots 0 0 0 1 2 2 2
  spline S194 degree 2 poles (24.964, -17.4961) (24.8174, -17.2877) (24.6861, -16.6753) (24.6861, -16.2637) knots 0 0 0 1 2 2 2
  spline S195 degree 2 poles (24.6861, -16.2637) (24.6861, -15.8417) (24.8174, -15.2448) (24.9666, -15.0286) knots 0 0 0 1 2 2 2
  spline S196 degree 2 poles (24.9666, -15.0286) (25.1158, -14.8177) (25.5867, -14.6118) (25.9109, -14.6118) knots 0 0 0 1 2 2 2
  spline S197 degree 2 poles (25.9109, -14.6118) (26.2531, -14.6118) (26.711, -14.828) (26.8577, -15.0415) knots 0 0 0 1 2 2 2
  spline S198 degree 2 poles (26.8577, -15.0415) (27.0018, -15.2499) (27.133, -15.8649) (27.133, -16.2637) knots 0 0 0 1 2 2 2
  spline S199 degree 2 poles (26.3328, -16.2637) (26.3328, -15.6745) (26.1399, -15.1985) (25.9109, -15.1985) knots 0 0 0 1 2 2 2
  spline S200 degree 2 poles (25.9109, -15.1985) (25.6819, -15.1985) (25.4863, -15.6745) (25.4863, -16.2662) knots 0 0 0 1 2 2 2
  spline S201 degree 2 poles (25.4863, -16.2662) (25.4863, -16.8477) (25.6819, -17.3314) (25.9109, -17.3314) knots 0 0 0 1 2 2 2
  spline S202 degree 2 poles (25.9109, -17.3314) (26.1373, -17.3314) (26.3328, -16.8477) (26.3328, -16.2637) knots 0 0 0 1 2 2 2
  line L167 (29.9555, -17.8512) -> (27.6219, -17.8512)
  line L168 (27.6219, -17.8512) -> (27.6219, -17.334)
  spline S203 degree 2 poles (27.6219, -17.334) (27.9177, -17.0973) (28.3912, -16.6805) (28.5687, -16.4926) knots 0 0 0 1 2 2 2
  spline S204 degree 2 poles (28.5687, -16.4926) (28.8028, -16.2482) (29.0112, -15.8751) (29.0112, -15.6796) knots 0 0 0 1 2 2 2
  spline S205 degree 2 poles (29.0112, -15.6796) (29.0112, -15.4583) (28.7462, -15.2216) (28.5095, -15.2216) knots 0 0 0 1 2 2 2
  spline S206 degree 2 poles (28.5095, -15.2216) (28.3886, -15.2216) (28.1725, -15.2808) (28.0618, -15.3271) knots 0 0 0 1 2 2 2
  spline S207 degree 2 poles (28.0618, -15.3271) (27.9538, -15.376) (27.7994, -15.4789) (27.7608, -15.5046) knots 0 0 0 1 2 2 2
  line L169 (27.7608, -15.5046) -> (27.699, -15.5046)
  line L170 (27.699, -15.5046) -> (27.699, -14.8125)
  spline S208 degree 2 poles (27.699, -14.8125) (27.8328, -14.7482) (28.404, -14.6144) (28.669, -14.6144) knots 0 0 0 1 2 2 2
  spline S209 degree 2 poles (28.669, -14.6144) (29.2351, -14.6144) (29.8166, -15.1187) (29.8166, -15.5741) knots 0 0 0 1 2 2 2
  spline S210 degree 2 poles (29.8166, -15.5741) (29.8166, -15.8546) (29.5516, -16.3949) (29.2454, -16.7036) knots 0 0 0 1 2 2 2
  spline S211 degree 2 poles (29.2454, -16.7036) (29.0524, -16.894) (28.6896, -17.1899) (28.6099, -17.2517) knots 0 0 0 1 2 2 2
  line L171 (28.6099, -17.2517) -> (29.9555, -17.2517)
  line L172 (29.9555, -17.2517) -> (29.9555, -17.8512)
  spline S212 degree 2 poles (32.7188, -16.7705) (32.7188, -17.2722) (32.0833, -17.9181) (31.5276, -17.9181) knots 0 0 0 1 2 2 2
  spline S213 degree 2 poles (31.5276, -17.9181) (31.2497, -17.9181) (30.8149, -17.7585) (30.6631, -17.6016) knots 0 0 0 1 2 2 2
  spline S214 degree 2 poles (30.6631, -17.6016) (30.483, -17.4189) (30.29, -16.84) (30.29, -16.436) knots 0 0 0 1 2 2 2
  spline S215 degree 2 poles (30.29, -16.436) (30.29, -16.0192) (30.4701, -15.3708) (30.6734, -15.1213) knots 0 0 0 1 2 2 2
  spline S216 degree 2 poles (30.6734, -15.1213) (30.8663, -14.8846) (31.4941, -14.617) (31.9238, -14.617) knots 0 0 0 1 2 2 2
  spline S217 degree 2 poles (31.9238, -14.617) (32.0808, -14.617) (32.3947, -14.6581) (32.4513, -14.671) knots 0 0 0 1 2 2 2
  line L173 (32.4513, -14.671) -> (32.4513, -15.2937)
  line L174 (32.4513, -15.2937) -> (32.3947, -15.2937)
  spline S218 degree 2 poles (32.3947, -15.2937) (32.338, -15.2654) (32.0808, -15.1959) (31.9161, -15.1959) knots 0 0 0 1 2 2 2
  spline S219 degree 2 poles (31.9161, -15.1959) (31.543, -15.1959) (31.1365, -15.5895) (31.0876, -15.9549) knots 0 0 0 1 2 2 2
  spline S220 degree 2 poles (31.0876, -15.9549) (31.2446, -15.8546) (31.5662, -15.7362) (31.7694, -15.7362) knots 0 0 0 1 2 2 2
  spline S221 degree 2 poles (31.7694, -15.7362) (31.9418, -15.7362) (32.2428, -15.8288) (32.3586, -15.9163) knots 0 0 0 1 2 2 2
  spline S222 degree 2 poles (32.3586, -15.9163) (32.5233, -16.0424) (32.7188, -16.4515) (32.7188, -16.7705) knots 0 0 0 1 2 2 2
  spline S223 degree 2 poles (31.79, -17.2491) (31.8518, -17.1719) (31.9187, -16.9918) (31.9187, -16.8091) knots 0 0 0 1 2 2 2
  spline S224 degree 2 poles (31.9187, -16.8091) (31.9187, -16.6547) (31.8415, -16.4541) (31.772, -16.3949) knots 0 0 0 1 2 2 2
  spline S225 degree 2 poles (31.772, -16.3949) (31.7, -16.3331) (31.5224, -16.2894) (31.4221, -16.2894) knots 0 0 0 1 2 2 2
  spline S226 degree 2 poles (31.4221, -16.2894) (31.3372, -16.2894) (31.1622, -16.3331) (31.085, -16.364) knots 0 0 0 1 2 2 2
  spline S227 degree 2 poles (31.085, -16.364) (31.085, -16.3846) (31.0799, -16.4824) (31.0799, -16.557) knots 0 0 0 1 2 2 2
  spline S228 degree 2 poles (31.0799, -16.557) (31.0799, -16.8323) (31.1751, -17.1642) (31.2497, -17.2491) knots 0 0 0 1 2 2 2
  spline S229 degree 2 poles (31.2497, -17.2491) (31.3037, -17.3186) (31.4478, -17.3777) (31.525, -17.3777) knots 0 0 0 1 2 2 2
  spline S230 degree 2 poles (31.525, -17.3777) (31.5893, -17.3777) (31.7386, -17.3134) (31.79, -17.2491) knots 0 0 0 1 2 2 2
  point P0 (22, -11.35)
  point P1 (51.9257, -11.35)
  point P2 (22, -11.35)
  point P3 (22, -5.0636)
  dimension "d0" = 22.7
  dimension "d1" = 55
  constraints: 6 midpoint, 2 end point, 1 horizontal alignment, 1 vertical alignment, 2 other
extrude "Text" cut sketch "Sketch8" against normal blind 1 contours S22 S23 S24 L53 L54 S25 S26 S27 L5 | L5 S27 S28 S29 S30 S21 S22 | S30 S31 S32 L55 L56 S33 S34 S21 L5 | L121 L122 S113 S114 S111 S112 L118 L119 L5 | L5 L119 L120 L121 | L8 L9 L10 L11 L12 L13 L14 L15 L16 L17 L18 L19 | L20 L21 L22 L23 L24 L25 L26 | S0 S1 S2 L27 L28 S3 S4 S5 S6 L29 L30 S7 S8 | L32 L33 S11 S12 S13 L34 L35 L36 L37 L38 S14 S15 L39 | S16 L40 L41 L42 L43 L44 L45 L46 L47 L48 L49 L50 S17 S18 S19 L51 L52 S20 | S35 S36 S37 S38 S39 L57 S40 S41 L58 L59 S42 S43 L60 L61 L62 | L64 S48 S49 S50 L65 L66 L67 S51 S52 S53 L68 L69 L70 L71 L72 S54 S55 S56 S57 S58 L73 L74 | S59 S60 S61 L75 L76 S62 S63 S64 S65 L77 L78 S66 S67 | L80 S70 S71 L81 L82 L83 L84 L85 S72 S73 S74 L86 | S75 S76 S77 S78 S79 L87 S80 S81 L88 L89 S82 S83 L90 L91 L92 | L94 L95 L96 L97 L98 L99 L100 L101 | L105 L106 S88 S89 S90 S91 S92 S93 L107 L108 L109 | S98 S99 S100 S101 S102 L111 S103 S104 L112 L113 S105 S106 L114 L115 L116 | S119 L124 L125 L126 L127 L128 L129 L130 L131 L132 L133 L134 S120 S121 S122 L135 L136 S123 | S124 S125 S126 L137 L138 S127 S128 S129 S130 L139 L140 S131 S132 | L142 S135 S136 L143 L144 L145 L146 L147 S137 S138 S139 L148 | S140 S141 S142 S143 S144 S145 L149 L150 S146 S147 S148 S149 S150 | L151 L152 L153 L154 | S159 S160 S161 S162 S163 L155 S164 S165 S166 S167 S168 S169 L156 S170 | L157 L158 L159 L160 | L161 L162 S182 S183 S184 S185 S186 L163 L164 S187 S188 S189 S190 L165 L166 | S191 S192 S193 S194 S195 S196 S197 S198 | L167 L168 S203 S204 S205 S206 S207 L169 L170 S208 S209 S210 S211 L171 L172 | S212 S213 S214 S215 S216 S217 L173 L174 S218 S219 S220 S221 S222
sketch "Sketch9" plane through (-22, -11.35, -27.5) normal (0, -1, 0) x (1, 0, 0)
  line L0 (0, 55) -> (0, 0) projected
  line L1 (0, 55) -> (44, 55) projected
  line L2 (0, 53.6) -> (1.4283, 55)
  line L3 (1.4283, 55) -> (-5.5717, 62.1414)
  line L4 (-5.5717, 62.1414) -> (-7, 60.7414)
  line L5 (-7, 60.7414) -> (0, 53.6)
  circle A0 centre (-6.2859, 61.4414) radius 5
  circle A1 centre (22, 26) radius 3.375 projected
  line L6 (22, 55) -> (22, 26)
  line L7 (0, 27.5) -> (44, 27.5)
  line L8 (44, 53.6) -> (42.5717, 55)
  line L9 (42.5717, 55) -> (49.5717, 62.1414)
  line L10 (49.5717, 62.1414) -> (51, 60.7414)
  line L11 (51, 60.7414) -> (44, 53.6)
  circle A2 centre (50.2859, 61.4414) radius 5
  line L12 (0, 1.4) -> (1.4283, 0)
  line L13 (1.4283, 0) -> (-5.5717, -7.1414)
  line L14 (-5.5717, -7.1414) -> (-7, -5.7414)
  line L15 (-7, -5.7414) -> (0, 1.4)
  circle A3 centre (-6.2859, -6.4414) radius 5
  line L16 (44, 1.4) -> (42.5717, 0)
  line L17 (42.5717, 0) -> (49.5717, -7.1414)
  line L18 (49.5717, -7.1414) -> (51, -5.7414)
  line L19 (51, -5.7414) -> (44, 1.4)
  circle A4 centre (50.2859, -6.4414) radius 5
  point P0 (22, 27.5)
  point P1 (-3.5707, 57.2429)
  point P2 (-2.1424, 58.6429)
  point P3 (47.5707, 57.2429)
  point P4 (46.1424, 58.6429)
  point P5 (46.1424, -3.6429)
  point P6 (47.5707, -2.2429)
  point P7 (-3.5707, -2.2429)
  point P8 (-2.1424, -3.6429)
  dimension "d70" = 10
  dimension "d71" = 2
  dimension "d72" = 1.4
  dimension "d73" = 10
  constraints: 36 end point, 15 symmetric about line, 4 centre point, 3 midpoint, 2 parallel, 2 point on line, 1 horizontal, 1 perpendicular, 1 vertical, 3 other
  measures "d70" distance of L3.end L2.end
  measures "d71" distance of L2.start L2.end
  measures "d72" distance of L2.start L0.start
  measures "d73" diameter of A0
extrude "Micky Mouse Ears" add sketch "Sketch9" against normal blind 0.25 contours L1 L2 L0 | L0 L5 A0 L3 L1 | A0 L3 L4 L5 | L5 L4 L3 A0 | L8 L9 A2 L11 | A2 L9 L10 L11 | L11 L10 L9 A2 | L12 L13 A3 L15 | A3 L13 L14 L15 | L15 L14 L13 A3 | L19 A4 L17 L16 | A4 L17 L18 L19 | L19 L18 L17 A4
body "Solid1"
